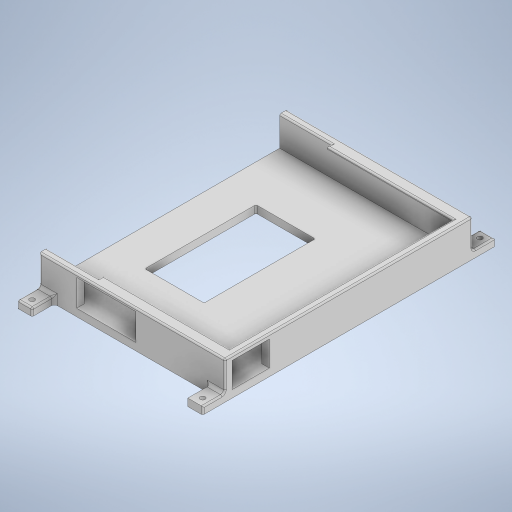
# Autodesk Inventor part: pccase
Saved by Autodesk Inventor 2023 (Build 270158000, 158)
## iProperties
Created: 2023-03-25
Part Number: pccase
Material: 一般
Document SubType Name: Modeling
Designer: fhbdh
Density: 1 g/cm^3
Appearance: 既定
Author: fhbdh
Autodesk Inventor part; units mm, degrees
ref_plane "YZ Plane" through (0, 0, 0) normal (1, 0, 0) x (0, 1, 0)
ref_plane "XZ Plane" through (0, 0, 0) normal (0, 1, 0) x (-1, 0, 0)
ref_plane "XY Plane" through (0, 0, 0) normal (0, 0, 1) x (1, 0, 0)
sketch "スケッチ1" plane through (0, 0, 0) normal (0, 1, 0) x (-1, 0, 0)
  line L0 (0, 0) -> (115, 0)
  line L1 (115, 0) -> (115, -157)
  line L2 (115, -157) -> (0, -157)
  line L3 (0, -157) -> (0, 0)
  line L4 (120, -162) -> (120, 5)
  line L5 (120, 5) -> (-5, 5)
  line L6 (-5, 5) -> (-5, -162)
  line L7 (-5, -162) -> (120, -162)
  dimension "d0" = 115
  dimension "d1" = 157
  dimension "d2" = 5
  constraints: 16 end point, 4 parallel, 2 perpendicular, 1 horizontal, 3 other
  measures "d0" distance of L1.end L2.end
  measures "d1" distance of L0.end L1.end
  measures "d2" distance between parallel lines of L1 L4
extrude "押し出し1" add sketch "スケッチ1" along normal blind 5 contours L0 L1 L2 L3 | L7 L6 L5 L4
sketch "スケッチ2" plane through (0, 5, 0) normal (0, 1, 0) x (1, 0, 0)
  line L0 (-120, -5) -> (5, -5) projected
  line L1 (5, -5) -> (5, 162) projected
  line L2 (5, 162) -> (-120, 162) projected
  line L3 (-120, 162) -> (-120, -5) projected
  line L4 (-115, 0) -> (0, 0)
  line L5 (0, 0) -> (0, 157)
  line L6 (0, 157) -> (-115, 157)
  line L7 (-115, 157) -> (-115, 0)
  line L8 (-115, 0) -> (-120, 0)
  line L9 (-120, 162) -> (-120, -5) projected
  line L10 (-115, 157) -> (-120, 157)
  point P0 (0, 0)
  dimension "d5" = 5
  constraints: 12 end point, 2 point on line, 1 parallel, 1 perpendicular, 3 other
  measures "d5" distance between parallel lines of L3 L7
extrude "押し出し2" add sketch "スケッチ2" along normal blind 20 contours L3 L8 L4 L5 L6 L10 L2 L1 L0
sketch "スケッチ3" plane through (0, 5, -157) normal (-1, 0, 0) x (0, 0, 1)
  line L0 (0, 0) -> (0, 20) projected
  line L1 (0, 20) -> (3, 20)
  line L2 (0, 20) -> (157, 20) projected
  line L3 (3, 20) -> (3, 18.5)
  line L4 (3, 18.5) -> (0, 17)
  line L5 (78.5, 20) -> (78.5, -5)
  line L6 (-5, -5) -> (162, -5) projected
  line L7 (157, 20) -> (154, 20)
  line L8 (154, 20) -> (154, 18.5)
  line L9 (154, 18.5) -> (157, 17)
  line L10 (157, 0) -> (0, 0) projected
  line L11 (157, 0) -> (157, 20) projected
  line L12 (0, 20) -> (157, 20) projected
  line L13 (0, 0) -> (0, 20) projected
  point P0 (157, -5)
  point P1 (157, 17)
  point P2 (154, 20)
  dimension "d8" = 3
  dimension "d9" = 1.5
  dimension "d10" = 1.5
  constraints: 14 end point, 3 symmetric about line, 2 midpoint, 2 point on line, 1 vertical
  measures "d8" distance of L0.end L1.end
  measures "d9" distance of L1.end L3.end
  measures "d10" vertical distance of L4.end L3.end
extrude "押し出し3" add sketch "スケッチ3" along normal blind 85 contours L0 L1 L3 L4 | L2 L11 L9 L8
sketch "スケッチ4" plane through (-120, 0, 5) normal (0, 0, 1) x (1, 0, 0)
  line L0 (120, 25) -> (35, 25) projected
  line L1 (65, 25) -> (25, 25)
  line L2 (25, 25) -> (25, 5)
  line L3 (25, 5) -> (65, 5)
  line L4 (65, 5) -> (65, 25)
  line L5 (0, 0) -> (0, 25) projected
  line L6 (0, 5) -> (120, 5) projected
  line L7 (25, 23) -> (65, 23)
  point P0 (120, 0)
  dimension "d13" = 65
  dimension "d14" = 40
  dimension "d15" = 0
  dimension "d16" = 2
  constraints: 10 end point, 3 point on line, 2 parallel, 2 perpendicular, 1 horizontal
  measures "d13" distance between parallel lines of L5 L4
  measures "d14" distance of L2.end L3.end
  measures "d15" distance between parallel lines of L6 L3
  measures "d16" distance between parallel lines of L0 L7
extrude "押し出し4" cut sketch "スケッチ4" against normal blind 10 contours L4 L3 L2 L7
sketch "スケッチ5" plane through (0, 0, 0) normal (0, -1, 0) x (1, 0, 0)
  line L0 (-95, -116) -> (-55, -116)
  line L1 (-55, -116) -> (-55, -41)
  line L2 (-55, -41) -> (-95, -41)
  line L3 (-95, -41) -> (-95, -116)
  line L4 (-120, -162) -> (-120, 5) projected
  point P0 (0, 0)
  point P1 (-120, -78.5)
  point P2 (-95, -78.5)
  dimension "d19" = 65
  dimension "d20" = 75
  dimension "d21" = 25
  dimension "d22" = 0
  constraints: 8 end point, 2 midpoint, 2 parallel, 1 horizontal, 1 perpendicular
  measures "d19" distance between parallel lines of L4 L1
  measures "d20" distance of L2.end L0.start
  measures "d21" distance between parallel lines of L4 L3
  measures "d22" vertical distance of point (-120, -78.5) point (-95, -78.5)
extrude "押し出し5" cut sketch "スケッチ5" against normal through all
sketch "スケッチ6" plane through (5, 0, 5) normal (1, 0, 0) x (0, 0, -1)
  line L0 (5, 5) -> (5, 22) projected
  line L1 (5, 5) -> (30, 5)
  line L2 (30, 5) -> (30, 22)
  line L3 (30, 22) -> (5, 22)
  line L4 (5, 22) -> (5, 5)
  point P0 (5, 0)
  dimension "d25" = 25
  dimension "d26" = 0
  constraints: 8 end point, 2 parallel, 1 horizontal, 1 perpendicular
  measures "d25" distance of L3.end L2.end
  measures "d26" distance from line of L0.end L3
extrude "押し出し6" cut sketch "スケッチ6" against normal up to surface (5 mm away)
sketch "スケッチ7" plane through (0, 0, 0) normal (0, -1, 0) x (1, 0, 0)
  circle A0 centre (-115, 15) radius 1.7
  circle A1 centre (0, 15) radius 1.7
  circle A2 centre (-115, -172) radius 1.7
  circle A3 centre (0, -172) radius 1.7
  line L0 (5, -162) -> (-120, -162) projected
  line L1 (-5, -162) -> (5, -162)
  line L2 (5, -162) -> (5, -177)
  line L3 (5, -177) -> (-5, -177)
  line L4 (-5, -177) -> (-5, -162)
  line L5 (-110, -162) -> (-120, -162)
  line L6 (-120, -162) -> (-120, -177)
  line L7 (-120, -177) -> (-110, -177)
  line L8 (-110, -177) -> (-110, -162)
  line L9 (-120, 5) -> (5, 5) projected
  line L10 (-120, 5) -> (-110, 5)
  line L11 (-110, 5) -> (-110, 20)
  line L12 (-110, 20) -> (-120, 20)
  line L13 (-120, 20) -> (-120, 5)
  line L14 (-5, 5) -> (5, 5)
  line L15 (5, 5) -> (5, 20)
  line L16 (5, 20) -> (-5, 20)
  line L17 (-5, 20) -> (-5, 5)
  line L18 (5, 5) -> (5, -162) projected
  line L19 (-120, -162) -> (-120, 5) projected
  circle A4 centre (120, -172) radius 1.7
  circle A5 centre (62.9804, -172) radius 1.525
  point P0 (0, 0)
  dimension "d29" = 3.4
  dimension "d30" = 3.4
  dimension "d31" = 3.4
  dimension "d32" = 3.4
  dimension "d33" = 5
  dimension "d34" = 5
  dimension "d35" = 5
  dimension "d36" = 5
  dimension "d37" = 5
  dimension "d38" = 5
  dimension "d39" = 5
  dimension "d40" = 5
  dimension "d41" = 5
  dimension "d42" = 5
  dimension "d43" = 5
  dimension "d44" = 5
  dimension "d45" = 10
  dimension "d46" = 10
  dimension "d47" = 10
  dimension "d48" = 10
  dimension "d56" = 0
  dimension "d57" = 0
  dimension "d60" = 57.0196
  dimension "d63" = 0
  dimension "d64" = 0
  constraints: 32 end point, 8 parallel, 6 centre point, 4 coincident, 4 horizontal, 4 perpendicular, 4 point on line
  measures "d29" diameter of A0
  measures "d30" diameter of A1
  measures "d31" diameter of A2
  measures "d32" diameter of A3
  measures "d33" distance from line of L12 point (-115, 15)
  measures "d34" distance from line of L11 point (-115, 15)
  measures "d35" distance from line of L13 point (-115, 15)
  measures "d36" distance from line of L15 point (0, 15)
  measures "d37" distance from line of L17 point (0, 15)
  measures "d38" distance from line of L16 point (0, 15)
  measures "d39" distance from line of L8 point (-115, -172)
  measures "d40" distance from line of L6 point (-115, -172)
  measures "d41" distance from line of L7 point (-115, -172)
  measures "d42" distance from line of L4 point (0, -172)
  measures "d43" distance from line of L2 point (0, -172)
  measures "d44" distance from line of L3 point (0, -172)
  measures "d45" distance from line of L0 point (0, -172)
  measures "d46" distance from line of L0 point (-115, -172)
  measures "d47" distance from line of L9 A0.centre
  measures "d48" distance from line of L9 A1.centre
  measures "d56" distance from line of L9.end L15
  measures "d57" distance between parallel lines of L2 L18
  measures "d60" distance of A5.centre A4.centre
  measures "d63" distance between parallel lines of L19 L6
  measures "d64" distance from line of L9.start L13
extrude "押し出し7" add sketch "スケッチ7" against normal blind 5 contours L2 L3 L4 L0 | L9 L17 L16 L15 | L8 L7 L6 L0 | L9 L13 L12 L11
fillet "フィレット1" radius 2 8 edges at (-110, 2.5, 5) (-5, 2.5, 5) (-110, 2.5, -162) (-5, 2.5, -162) (0, 5, -162) (-115, 5, -162) (-115, 5, 5) (0, 5, 5)
fillet "フィレット2" radius 1 37 edges at (5, 5, 13.5) (5, 16, 5) (5, 2.5, 20) (-57.5, 25, 5) (-110, 2.5, 20) (-120, 2.5, 20) (-5, 2.5, -177) (-57.5, 25, -162) (5, 25, -78.5) (5, 5, -170.5) (5, 16, -162) (-5.5858, 5.5858, -162.5858) (-5, 5, -170.5) (0, 5, -177) (-115, 5, -177) (-109.4142, 5.5858, -162.5858) (-110, 5, -170.5) (-120, 2.5, -177) (-110, 2.5, -177) (-120, 16, -162) (-120, 5, -170.5) (-120, 5, 13.5) (-120, 16, 5) (-109.4142, 5.5858, 5.5858) (-110, 5, 13.5) (-115, 5, 20) (-42.5, 25, -3) (-102.5, 25, 0) (0, 25, -78.5) (-42.5, 25, -154) (-102.5, 25, -157) (-85, 25, -155.5) (-85, 25, -1.5) (-95, 2.5, -41) (-55, 2.5, -41) (-55, 2.5, -116) (-95, 2.5, -116)
